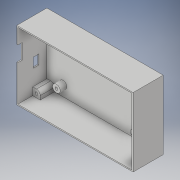
# Autodesk Inventor part: case_bottom
Saved by Autodesk Inventor 2019 (Build 230136000, 136)
## iProperties
Created: 2019-03-26
Part Number: case_bottom
Material: Generic
Document SubType Name: Modeling
Designer: janza
Density: 1 g/cm^3
Appearance: Default
Author: janza
## iProperties of the stored document case_bottom_3DPrint.ipt
Created: 2019-03-26
Part Number: case_bottom_3DPrint
Material: Generic
Document SubType Name: Modeling
Designer: janza
Density: 1 g/cm^3
Appearance: Default
Author: janza
Autodesk Inventor part; units mm, degrees
ref_plane "YZ Plane" through (0, 0, 0) normal (1, 0, 0) x (0, 1, 0)
ref_plane "XZ Plane" through (0, 0, 0) normal (0, 1, 0) x (-1, 0, 0)
ref_plane "XY Plane" through (0, 0, 0) normal (0, 0, 1) x (1, 0, 0)
sketch "zaklad" plane through (0, 0, 0) normal (0, 0, 1) x (1, 0, 0)
  line L0 (0, 0) -> (120, 0)
  line L1 (120, 0) -> (120, -70)
  line L2 (120, -70) -> (0, -70)
  line L3 (0, -70) -> (0, 0)
  dimension "d0" = 120
  dimension "d1" = 70
  constraints: 8 end point, 2 parallel, 1 horizontal, 1 perpendicular
  measures "d0" distance of L1.end L2.end
  measures "d1" distance of L0.end L1.end
extrude "Extrusion1" add sketch "zaklad" along normal blind 1.2
sketch "uchyt_pro_desku" plane through (0, 0, 1.2) normal (0, 0, 1) x (1, 0, 0)
  line L0 (0, 0) -> (0, -70) projected
  line L1 (0, -35) -> (120, -35)
  line L2 (120, -70) -> (120, 0) projected
  circle A0 centre (17, -59) radius 4
  circle A1 centre (17, -59) radius 1.5
  circle A2 centre (17, -11) radius 4
  circle A3 centre (17, -11) radius 1.5
  circle A4 centre (92.5, -11) radius 4
  circle A5 centre (92.5, -11) radius 1.5
  circle A6 centre (99, -59) radius 4
  circle A7 centre (99, -59) radius 1.5
  dimension "d4" = 8
  dimension "d5" = 17
  dimension "d6" = 24
  dimension "d7" = 3
  dimension "d8" = 8
  dimension "d9" = 75.5
  dimension "d10" = 3
  dimension "d11" = 8
  dimension "d12" = 82
  dimension "d13" = 3
  constraints: 8 centre point, 4 coincident, 2 end point, 2 midpoint, 2 symmetric about line, 2 other
  measures "d4" diameter of A0
  measures "d5" distance from line of L0 A0.centre
  measures "d6" distance from line of L1 A0.centre
  measures "d7" diameter of A1
  measures "d8" diameter of A4
  measures "d9" distance of A4.centre A2.centre
  measures "d10" diameter of A5
  measures "d11" diameter of A6
  measures "d12" distance of A0.centre A6.centre
  measures "d13" diameter of A7
extrude "Extrusion2" add sketch "uchyt_pro_desku" along normal blind 7
sketch "stena_RJ45" plane through (0, 0, 1.2) normal (0, 0, 1) x (1, 0, 0)
  line L0 (-1.2, -16) -> (0, -16)
  line L1 (0, -16) -> (0, -32.2)
  line L2 (0, -32.2) -> (-1.2, -32.2)
  line L3 (-1.2, -32.2) -> (-1.2, -16)
  circle A0 centre (17, -11) radius 4 projected
  line L4 (0, 0) -> (0, -70) projected
  dimension "d17" = 1.2
  dimension "d18" = 16.2
  dimension "d19" = 5
  dimension "d20" = 0
  constraints: 8 end point, 2 parallel, 1 coincident, 1 horizontal, 1 perpendicular
  measures "d17" distance of L1.end L2.end
  measures "d18" distance of L0.end L1.end
  measures "d19" distance from line of A0.centre L0
  measures "d20" distance between parallel lines of L4 L1
sketch "srouby_upevneni" plane through (0, 0, 1.2) normal (0, 0, 1) x (1, 0, 0)
  arc A0 (8, -66) -> (4, -62) centre (4, -66) ccw
  line L0 (0, -70) -> (120, -70) projected
  line L1 (0, 0) -> (0, -70) projected
  line L2 (8, -66) -> (8, -70)
  line L3 (4, -62) -> (0, -62)
  line L4 (0, -62) -> (0, -70)
  line L5 (8, -70) -> (0, -70)
  circle A1 centre (4, -66) radius 1.5
  line L6 (120, -70) -> (120, 0) projected
  line L7 (120, -35) -> (0, -35)
  line L8 (60, -35) -> (60, -22.3833)
  arc A2 (4, -8) -> (8, -4) centre (4, -4) ccw
  line L9 (8, -4) -> (8, 0)
  line L10 (4, -8) -> (0, -8)
  line L11 (0, -8) -> (0, 0)
  line L12 (8, 0) -> (0, 0)
  circle A3 centre (4, -4) radius 1.5
  arc A4 (116, -62) -> (112, -66) centre (116, -66) ccw
  line L13 (112, -66) -> (112, -70)
  line L14 (116, -62) -> (120, -62)
  line L15 (120, -62) -> (120, -70)
  line L16 (112, -70) -> (120, -70)
  circle A5 centre (116, -66) radius 1.5
  line L17 (112, -4) -> (112, 0)
  arc A6 (112, -4) -> (116, -8) centre (116, -4) ccw
  circle A7 centre (116, -4) radius 1.5
  line L18 (116, -8) -> (120, -8)
  line L19 (120, -8) -> (120, 0)
  line L20 (112, 0) -> (120, 0)
  dimension "d21" = 8
  dimension "d22" = 3
  constraints: 36 end point, 18 symmetric about line, 8 centre point, 8 point on circle, 4 coincident, 4 tangent, 3 midpoint, 3 perpendicular, 2 point on line, 1 collinear, 1 vertical, 6 other
  measures "d21" diameter of A0
  measures "d22" diameter of A1
sketch "steny" plane through (0, 0, 1.2) normal (0, 0, 1) x (1, 0, 0)
  line L0 (0, -32.2) -> (-1.2, -32.2) projected
  line L1 (-1.2, -16) -> (0, -16) projected
  line L2 (0, -32.2) -> (-1.2, -32.2)
  line L3 (-1.2, -32.2) -> (-1.2, -70)
  line L4 (-1.2, -70) -> (-1.2, -71.2)
  line L5 (-1.2, -71.2) -> (120, -71.2)
  line L6 (120, -71.2) -> (121.2, -71.2)
  line L7 (121.2, -71.2) -> (121.2, 0)
  line L8 (120, -70) -> (120, 0) projected
  line L9 (121.2, 0) -> (121.2, 1.2)
  line L10 (121.2, 1.2) -> (0, 1.2)
  line L11 (0, 0) -> (0, -70) projected
  line L12 (0, 1.2) -> (-1.2, 1.2)
  line L13 (-1.2, 1.2) -> (-1.2, -16)
  line L14 (0, -16) -> (-1.2, -16)
  line L15 (0, -16) -> (0, 0)
  line L16 (120, 0) -> (0, 0) projected
  line L17 (0, 0) -> (120, 0)
  line L18 (120, 0) -> (120, -70)
  line L19 (120, -70) -> (0, -70)
  line L20 (0, -70) -> (0, -32.2)
  dimension "d23" = 1.2
  dimension "d24" = 1.2
  dimension "d25" = 1.2
  dimension "d26" = 1.2
  constraints: 32 end point, 6 perpendicular, 5 point on line, 3 parallel, 1 collinear, 1 horizontal, 1 vertical
  measures "d23" distance of L3.end L4.end
  measures "d24" distance of L5.end L6.end
  measures "d25" distance of L7.end L9.end
  measures "d26" distance of L10.end L12.end
extrude "Extrusion3" add sketch "steny" along normal blind 30.5 and the other way blind 1.2 contours L11 L19 L8 L16 L1 L13 L12 L10 L9 L7 L6 L5 L4 L3 L0
extrude "Extrusion4" add sketch "stena_RJ45" along normal blind 26 and the other way blind 1.2 contours L0 L1 L2 L3
extrude "Extrusion5" add sketch "srouby_upevneni" along normal blind 15 contours L2 L0 L1 L3 A0 | L13 A4 L14 L6 L0 | L12 L9 A2 L10 L1 | L18 A6 L17 L20 L6
sketch "diry" plane through (0, 0, 1.2) normal (0, 0, 1) x (1, 0, 0)
  circle A0 centre (4, -4) radius 1.5 projected
  circle A1 centre (116, -4) radius 1.5 projected
  circle A2 centre (116, -66) radius 1.5 projected
  circle A3 centre (4, -66) radius 1.5 projected
  point P0 (0, 0)
  constraints: 4 coincident
hole "Hole1" at (4, -4, 1.2) at (116, -4, 1.2) at (116, -66, 1.2) at (4, -66, 1.2) direction (0, 0, -1) diameter 3 end through all
sketch "dira_USB" plane through (-1.2, -71.2, 0) normal (-1, 0, 0) x (0, 0, 1)
  line L0 (15.7, 36) -> (9.7, 36)
  line L1 (9.7, 36) -> (9.7, 26)
  line L2 (9.7, 26) -> (15.7, 26)
  line L3 (15.7, 26) -> (15.7, 36)
  line L4 (27.2, 39) -> (31.7, 39) projected
  line L5 (27.2, 55.2) -> (27.2, 39) projected
  point P0 (0, 71.2)
  dimension "d44" = 6
  dimension "d45" = 10
  dimension "d46" = 3
  dimension "d47" = 11.5
  constraints: 8 end point, 2 parallel, 1 horizontal, 1 perpendicular
  measures "d44" distance of L2.end L1.end
  measures "d45" distance of L1.end L0.end
  measures "d46" distance between parallel lines of L0 L4
  measures "d47" distance between parallel lines of L3 L5
extrude "Extrusion6" cut sketch "dira_USB" against normal blind 5
body "Solid1"
